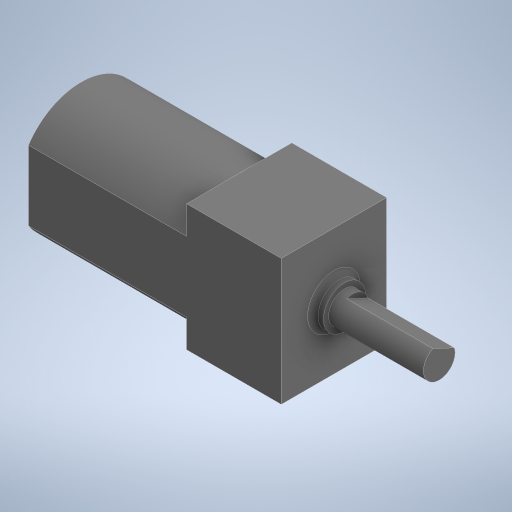
# Autodesk Inventor part: GA12-N20 Motor_finalV
Saved by Autodesk Inventor 2023.2 (Build 272271030, 271C)
## iProperties
Created: 2023-03-18
Part Number: GA12-N20 Motor_finalV
Material: Všeobecné
Document SubType Name: Modeling
Designer: Simak
Density: 1 g/cm^3
Appearance: Šedá
Author: Simak
Autodesk Inventor part; units mm, degrees
ref_plane "YZ Plane" through (0, 0, 0) normal (1, 0, 0) x (0, 1, 0)
ref_plane "XZ Plane" through (0, 0, 0) normal (0, 1, 0) x (-1, 0, 0)
ref_plane "Pracovní rovina2" through (10, 0, 0) normal (1, 0, 0) x (0, 0, -1)
sketch "Náčrt1" plane through (10, 0, 0) normal (1, 0, 0) x (0, 0, -1)
  arc A0 (-3.3166, 5) -> (-3.3166, -5) centre (0, 0) ccw projected
  line L0 (3.3166, 5) -> (-3.3166, 5) projected
  arc A1 (3.3166, -5) -> (3.3166, 5) centre (0, 0) ccw projected
  line L1 (-3.3166, -5) -> (3.3166, -5) projected
  point P0 (0, 0)
extrude "Vysunutí1" add sketch "Náčrt1" along normal blind 15
sketch "Náčrt2" plane through (25, 0, 0) normal (1, 0, 0) x (0, 0, -1)
  line L0 (-6, 5) -> (-6, -5) projected
  line L1 (6, 5) -> (-6, 5) projected
  line L2 (6, 5) -> (6, -5) projected
  line L3 (-6, -5) -> (6, -5) projected
  point P0 (0, 0)
extrude "Vysunutí2" add sketch "Náčrt2" along normal blind 9
sketch "Náčrt3" plane through (34, 0, 0) normal (1, 0, 0) x (0, 0, -1)
  arc A0 (-1.3795, -0.589) -> (-0.4321, 1.4364) centre (0, 0) ccw projected
  line L0 (-1.3795, -0.589) -> (-0.4321, 1.4364) projected
  circle A1 centre (0, 0) radius 2 projected
  arc A2 (-0.4321, 1.4364) -> (-1.3795, -0.589) centre (0, 0) ccw projected
extrude "Vysunutí3" add sketch "Náčrt3" along normal blind 1
extrude "Vysunutí4" add sketch "Náčrt3" along normal blind 10 contours L0 A0
extrude "Vysunutí5" add sketch "Náčrt3" along normal blind 1.8 contours A2 L0
sketch "Náčrt4" plane through (10, 0, 0) normal (-1, 0, 0) x (0, 0, 1)
  circle A0 centre (0, 0) radius 2.5
  dimension "d12" = 5
  constraints: 1 centre point, 1 coincident
  measures "d12" diameter of A0
extrude "Vysunutí6" add sketch "Náčrt4" along normal blind 0.8
fillet "Zaoblení2" radius 0.5 1 edges at (34, 0, 2)
